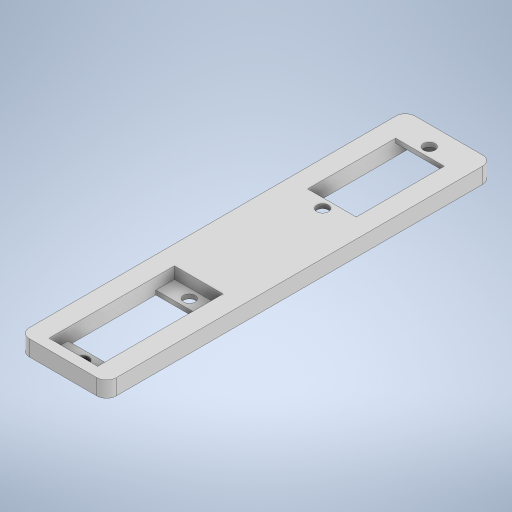
# Autodesk Inventor part: arm_medium_part
Saved by Autodesk Inventor 2023 (Build 270158000, 158)
## iProperties
Created: 2023-02-22
Part Number: arm_medium_part
Material: Ogólny
Document SubType Name: Modeling
Designer: kamil
Density: 1 g/cm^3
Appearance: Domyślna
Author: kamil
Autodesk Inventor part; units mm, degrees
ref_plane "YZ Plane" through (0, 0, 0) normal (1, 0, 0) x (0, 1, 0)
ref_plane "XZ Plane" through (0, 0, 0) normal (0, 1, 0) x (-1, 0, 0)
ref_plane "XY Plane" through (0, 0, 0) normal (0, 0, 1) x (1, 0, 0)
sketch "Szkic1" plane through (0, 0, 0) normal (0, 1, 0) x (-1, 0, 0)
  line L0 (8.75, 50) -> (-8.75, 50)
  line L1 (-11.25, 47.5) -> (-11.25, -47.5)
  line L2 (-8.75, -50) -> (8.75, -50)
  line L3 (11.25, -47.5) -> (11.25, 47.5)
  line L4 (-11.25, 50) -> (11.25, -50)
  line L5 (-11.25, -50) -> (11.25, 50)
  arc A0 (11.25, 47.5) -> (8.75, 50) centre (8.75, 47.5) ccw
  arc A1 (-8.75, 50) -> (-11.25, 47.5) centre (-8.75, 47.5) ccw
  arc A2 (-11.25, -47.5) -> (-8.75, -50) centre (-8.75, -47.5) ccw
  arc A3 (8.75, -50) -> (11.25, -47.5) centre (8.75, -47.5) ccw
  point P0 (0, 0)
  point P1 (0, 0)
  dimension "d0" = 22.5
  dimension "d1" = 100
  dimension "d2" = 2.5
  constraints: 12 end point, 8 point on circle, 8 point on line, 8 tangent, 4 centre point, 3 equal radius, 2 parallel, 1 coincident, 1 horizontal, 1 midpoint, 1 perpendicular
  measures "d0" distance of L4.end L5.start
  measures "d1" distance of L5.start L4.start
  measures "d2" radius of A0
extrude "Wyciągnięcie proste1" add sketch "Szkic1" along normal blind 4.1
sketch "Szkic2" plane through (0, 4.1, 0) normal (0, 1, 0) x (1, 0, 0)
  line L0 (-6.3, -42.5) -> (6.3, -42.5)
  line L1 (6.3, -42.5) -> (6.3, -19.7)
  line L2 (6.3, -19.7) -> (-6.3, -19.7)
  line L3 (-6.3, -19.7) -> (-6.3, -42.5)
  line L4 (-8.75, -50) -> (8.75, -50) projected
  line L5 (11.25, -47.5) -> (11.25, 47.5) projected
  line L6 (-6.3, 19.7) -> (6.3, 19.7)
  line L7 (6.3, 19.7) -> (6.3, 42.5)
  line L8 (6.3, 42.5) -> (-6.3, 42.5)
  line L9 (-6.3, 42.5) -> (-6.3, 19.7)
  line L10 (-15.75, 0) -> (15.75, 0) projected
  point P0 (0, 0)
  point P1 (0, -42.5)
  dimension "d5" = 12.6
  dimension "d6" = 22.8
  dimension "d7" = 7.5
  dimension "d8" = 11.25
  constraints: 16 end point, 4 parallel, 2 equal length, 2 horizontal, 2 perpendicular, 1 midpoint, 2 other
  measures "d5" distance of L2.end L1.end
  measures "d6" distance of L1.end L0.end
  measures "d7" distance between parallel lines of L4 L0
  measures "d8" distance from line of L5 point (0, -42.5)
extrude "Wyciągnięcie proste2" cut sketch "Szkic2" against normal blind 4.1
sketch "Szkic4" plane through (0, 4.1, 0) normal (0, 1, 0) x (1, 0, 0)
  line L0 (-6.3, -47.35) -> (6.3, -47.35)
  line L1 (6.3, -47.35) -> (6.3, -14.85)
  line L2 (6.3, -14.85) -> (-6.3, -14.85)
  line L3 (-6.3, -14.85) -> (-6.3, -47.35)
  line L4 (6.3, -42.5) -> (-6.3, -42.5) projected
  line L5 (-6.3, -19.7) -> (6.3, -19.7) projected
  point P0 (0, 0)
  dimension "d11" = 4.85
  dimension "d12" = 4.85
  constraints: 8 end point, 2 parallel, 1 horizontal, 1 perpendicular
  measures "d11" distance from line of L4 L0.start
  measures "d12" distance from line of L5 L2.end
extrude "Wyciągnięcie proste3" cut sketch "Szkic4" against normal blind 3 contours L3 L4 L1 L0 | L3 L2 L1 L5
sketch "Szkic5" plane through (0, 1.1, 0) normal (0, 1, 0) x (1, 0, 0)
  circle A0 centre (0, -44.925) radius 1.5
  circle A1 centre (0, -17.275) radius 1.5
  circle A2 centre (0, 17.275) radius 1.5
  circle A3 centre (0, 44.925) radius 1.5
  line L0 (-6.3, -42.5) -> (6.3, -42.5) projected
  line L1 (6.3, -19.7) -> (-6.3, -19.7) projected
  line L2 (-6.3, 19.7) -> (6.3, 19.7) projected
  line L3 (6.3, 42.5) -> (-6.3, 42.5) projected
  point P0 (0, 0)
  point P1 (0, -42.5)
  point P2 (0, -19.7)
  point P3 (0, 19.7)
  point P4 (0, 42.5)
  dimension "d17" = 3
  dimension "d18" = 3
  dimension "d19" = 3
  dimension "d20" = 3
  dimension "d21" = 2.425
  dimension "d22" = 2.425
  dimension "d23" = 2.425
  dimension "d24" = 2.425
  constraints: 4 centre point, 4 midpoint
  measures "d17" diameter of A0
  measures "d18" diameter of A1
  measures "d19" diameter of A2
  measures "d20" diameter of A3
  measures "d21" distance of A0.centre point (0, -42.5)
  measures "d22" distance of point (0, -19.7) A1.centre
  measures "d23" distance of point (0, 19.7) A2.centre
  measures "d24" distance of A3.centre point (0, 42.5)
extrude "Wyciągnięcie proste4" cut sketch "Szkic5" against normal blind 3
sketch "Szkic6" plane through (0, 0, 0) normal (0, -1, 0) x (1, 0, 0)
  line L0 (-6.3, -19.7) -> (6.3, -19.7)
  line L1 (6.3, -19.7) -> (6.3, -14.85)
  line L2 (6.3, -14.85) -> (-6.3, -14.85)
  line L3 (-6.3, -14.85) -> (-6.3, -19.7)
  line L4 (-6.3, -47.35) -> (6.3, -47.35)
  line L5 (6.3, -47.35) -> (6.3, -42.5)
  line L6 (6.3, -42.5) -> (-6.3, -42.5)
  line L7 (-6.3, -42.5) -> (-6.3, -47.35)
  point P0 (0, 0)
  dimension "d27" = 4.85
  dimension "d28" = 4.85
  constraints: 16 end point, 4 parallel, 3 coincident, 2 horizontal, 2 perpendicular
  measures "d27" distance of L1.end L0.end
  measures "d28" distance of L4.end L5.end
extrude "Wyciągnięcie proste5" cut sketch "Szkic6" against normal blind 3
sketch "Szkic7" plane through (0, 3, 0) normal (0, -1, 0) x (1, 0, 0)
  circle A0 centre (0, -44.925) radius 1.5
  circle A1 centre (0, -17.275) radius 1.5
  line L0 (6.3, -19.7) -> (-6.3, -19.7) projected
  line L1 (-6.3, -42.5) -> (6.3, -42.5) projected
  point P0 (0, 0)
  point P1 (0, -19.7)
  dimension "d31" = 3
  dimension "d32" = 3
  dimension "d33" = 2.425
  dimension "d34" = 2.425
  constraints: 2 centre point, 1 midpoint
  measures "d31" diameter of A0
  measures "d32" diameter of A1
  measures "d33" distance of point (0, -19.7) A1.centre
  measures "d34" distance from line of L1 A0.centre
extrude "Wyciągnięcie proste6" cut sketch "Szkic7" against normal blind 3
